Autodesk Fusion 360 part; units mm, degrees
(part 2 of 2)
  spline S168 degree 3 poles (-19.8203, 34.3524) (-19.856, 34.4918) (-19.8914, 34.6421) (-19.9257, 34.8034) knots 0 0 0 0 1 1 1 1
  spline S169 degree 3 poles (-19.9257, 34.8034) (-20.0542, 35.4074) (-20.1673, 36.1627) (-20.2205, 37.0718) knots 0 0 0 0 1 1 1 1
  arc A170 (-19.5901, 37.4087) -> (-20.2205, 37.0718) centre (0, 0) ccw
  spline S170 degree 3 poles (-19.5901, 37.4087) (-18.8638, 36.8595) (-18.2986, 36.3458) (-17.8679, 35.9033) knots 0 0 0 0 1 1 1 1
  spline S171 degree 3 poles (-17.8679, 35.9033) (-17.7528, 35.7852) (-17.6475, 35.6723) (-17.5514, 35.5652) knots 0 0 0 0 1 1 1 1
  arc A171 (-17.5514, 35.5652) -> (-17.0802, 35.472) centre (-17.2537, 35.8324) ccw
  arc A172 (-16.5847, 35.7064) -> (-17.0802, 35.472) centre (0, 0) ccw
  arc A173 (-16.5847, 35.7064) -> (-16.3578, 36.1297) centre (-16.7532, 36.0692) ccw
  spline S172 degree 3 poles (-16.3578, 36.1297) (-16.3796, 36.272) (-16.4, 36.425) (-16.4184, 36.5889) knots 0 0 0 0 1 1 1 1
  spline S173 degree 3 poles (-16.4184, 36.5889) (-16.4871, 37.2025) (-16.5257, 37.9653) (-16.4895, 38.8752) knots 0 0 0 0 1 1 1 1
  arc A174 (-15.8291, 39.1488) -> (-16.4895, 38.8752) centre (0, 0) ccw
  spline S174 degree 3 poles (-15.8291, 39.1488) (-15.1601, 38.531) (-14.648, 37.9643) (-14.2627, 37.4818) knots 0 0 0 0 1 1 1 1
  spline S175 degree 3 poles (-14.2627, 37.4818) (-14.1598, 37.353) (-14.0661, 37.2303) (-13.9809, 37.1143) knots 0 0 0 0 1 1 1 1
  arc A175 (-13.9809, 37.1143) -> (-13.5211, 36.9754) centre (-13.6585, 37.351) ccw
  arc A176 (-13.005, 37.16) -> (-13.5211, 36.9754) centre (0, 0) ccw
  arc A177 (-13.005, 37.16) -> (-12.7377, 37.5591) centre (-13.1371, 37.5376) ccw
  spline S176 degree 3 poles (-12.7377, 37.5591) (-12.7454, 37.7028) (-12.7508, 37.8571) (-12.753, 38.022) knots 0 0 0 0 1 1 1 1
  spline S177 degree 3 poles (-12.753, 38.022) (-12.7612, 38.6394) (-12.7248, 39.4023) (-12.5997, 40.3043) knots 0 0 0 0 1 1 1 1
  arc A178 (-11.9156, 40.5118) -> (-12.5997, 40.3043) centre (0, 0) ccw
  spline S178 degree 3 poles (-11.9156, 40.5118) (-11.3105, 39.8314) (-10.8563, 39.2173) (-10.5202, 38.6993) knots 0 0 0 0 1 1 1 1
  spline S179 degree 3 poles (-10.5202, 38.6993) (-10.4304, 38.561) (-10.3491, 38.4297) (-10.2757, 38.3059) knots 0 0 0 0 1 1 1 1
  arc A179 (-10.2757, 38.3059) -> (-9.8318, 38.1226) centre (-9.9317, 38.5099) ccw
  arc A180 (-9.3, 38.2558) -> (-9.8318, 38.1226) centre (0, 0) ccw
  arc A181 (-9.3, 38.2558) -> (-8.9949, 38.6267) centre (-9.3945, 38.6445) ccw
  spline S180 degree 3 poles (-8.9949, 38.6267) (-8.9885, 38.7705) (-8.9788, 38.9246) (-8.9648, 39.0889) knots 0 0 0 0 1 1 1 1
  spline S181 degree 3 poles (-8.9648, 39.0889) (-8.9125, 39.7042) (-8.8015, 40.4598) (-8.5885, 41.3452) knots 0 0 0 0 1 1 1 1
  arc A182 (-7.8874, 41.4846) -> (-8.5885, 41.3452) centre (0, 0) ccw
  spline S182 degree 3 poles (-7.8874, 41.4846) (-7.3518, 40.7482) (-6.9601, 40.0925) (-6.6763, 39.5441) knots 0 0 0 0 1 1 1 1
  spline S183 degree 3 poles (-6.6763, 39.5441) (-6.6005, 39.3977) (-6.5325, 39.259) (-6.4716, 39.1286) knots 0 0 0 0 1 1 1 1
  arc A183 (-6.4716, 39.1286) -> (-6.0478, 38.9027) centre (-6.1092, 39.298) ccw
  arc A184 (-5.5055, 38.9832) -> (-6.0478, 38.9027) centre (0, 0) ccw
  arc A185 (-5.5055, 38.9832) -> (-5.1655, 39.3224) centre (-5.5615, 39.3792) ccw
  spline S184 degree 3 poles (-5.1655, 39.3224) (-5.1451, 39.4649) (-5.1202, 39.6173) (-5.0902, 39.7794) knots 0 0 0 0 1 1 1 1
  spline S185 degree 3 poles (-5.0902, 39.7794) (-4.9779, 40.3866) (-4.7933, 41.1277) (-4.4946, 41.9879) knots 0 0 0 0 1 1 1 1
  arc A186 (-3.7832, 42.058) -> (-4.4946, 41.9879) centre (0, 0) ccw
  spline S186 degree 3 poles (-3.7832, 42.058) (-3.3224, 41.2726) (-2.9968, 40.5817) (-2.7682, 40.0081) knots 0 0 0 0 1 1 1 1
  spline S187 degree 3 poles (-2.7682, 40.0081) (-2.7071, 39.8549) (-2.653, 39.7103) (-2.6051, 39.5746) knots 0 0 0 0 1 1 1 1
  arc A187 (-2.6051, 39.5746) -> (-2.2055, 39.3082) centre (-2.2279, 39.7076) ccw
  arc A188 (-1.658, 39.3351) -> (-2.2055, 39.3082) centre (0, 0) ccw
  arc A189 (-1.658, 39.3351) -> (-1.2864, 39.6393) centre (-1.6748, 39.7347) ccw
  spline S188 degree 3 poles (-1.2864, 39.6393) (-1.2521, 39.7791) (-1.2124, 39.9284) (-1.1666, 40.0868) knots 0 0 0 0 1 1 1 1
  spline S189 degree 3 poles (-1.1666, 40.0868) (-0.9953, 40.68) (-0.739, 41.3995) (-0.3574, 42.2263) knots 0 0 0 0 1 1 1 1
  arc A190 (0.3574, 42.2263) -> (-0.3574, 42.2263) centre (0, 0) ccw
  spline S190 degree 3 poles (0.3574, 42.2263) (0.739, 41.3995) (0.9953, 40.68) (1.1666, 40.0868) knots 0 0 0 0 1 1 1 1
  spline S191 degree 3 poles (1.1666, 40.0868) (1.2124, 39.9284) (1.2521, 39.7791) (1.2864, 39.6393) knots 0 0 0 0 1 1 1 1
  arc A191 (1.2864, 39.6393) -> (1.658, 39.3351) centre (1.6748, 39.7347) ccw
  arc A192 (2.2055, 39.3082) -> (1.658, 39.3351) centre (0, 0) ccw
  arc A193 (2.2055, 39.3082) -> (2.6051, 39.5746) centre (2.2279, 39.7076) ccw
  spline S192 degree 3 poles (2.6051, 39.5746) (2.653, 39.7103) (2.7071, 39.8549) (2.7682, 40.0081) knots 0 0 0 0 1 1 1 1
  spline S193 degree 3 poles (2.7682, 40.0081) (2.9968, 40.5817) (3.3224, 41.2726) (3.7832, 42.058) knots 0 0 0 0 1 1 1 1
  arc A194 (4.4946, 41.9879) -> (3.7832, 42.058) centre (0, 0) ccw
  spline S194 degree 3 poles (4.4946, 41.9879) (4.7933, 41.1277) (4.9779, 40.3866) (5.0902, 39.7794) knots 0 0 0 0 1 1 1 1
  spline S195 degree 3 poles (5.0902, 39.7794) (5.1202, 39.6173) (5.1451, 39.4649) (5.1655, 39.3224) knots 0 0 0 0 1 1 1 1
  arc A195 (5.1655, 39.3224) -> (5.5055, 38.9832) centre (5.5615, 39.3792) ccw
  arc A196 (6.0478, 38.9027) -> (5.5055, 38.9832) centre (0, 0) ccw
  arc A197 (6.0478, 38.9027) -> (6.4716, 39.1286) centre (6.1092, 39.298) ccw
  spline S196 degree 3 poles (6.4716, 39.1286) (6.5325, 39.259) (6.6005, 39.3977) (6.6763, 39.5441) knots 0 0 0 0 1 1 1 1
  spline S197 degree 3 poles (6.6763, 39.5441) (6.9601, 40.0925) (7.3518, 40.7482) (7.8874, 41.4846) knots 0 0 0 0 1 1 1 1
  arc A198 (8.5885, 41.3452) -> (7.8874, 41.4846) centre (0, 0) ccw
  spline S198 degree 3 poles (8.5885, 41.3452) (8.8015, 40.4598) (8.9125, 39.7042) (8.9648, 39.0889) knots 0 0 0 0 1 1 1 1
  spline S199 degree 3 poles (8.9648, 39.0889) (8.9788, 38.9246) (8.9885, 38.7705) (8.9949, 38.6267) knots 0 0 0 0 1 1 1 1
  arc A199 (8.9949, 38.6267) -> (9.3, 38.2558) centre (9.3945, 38.6445) ccw
  arc A200 (9.8318, 38.1226) -> (9.3, 38.2558) centre (0, 0) ccw
  arc A201 (9.8318, 38.1226) -> (10.2757, 38.3059) centre (9.9317, 38.5099) ccw
  spline S200 degree 3 poles (10.2757, 38.3059) (10.3491, 38.4297) (10.4304, 38.561) (10.5202, 38.6993) knots 0 0 0 0 1 1 1 1
  spline S201 degree 3 poles (10.5202, 38.6993) (10.8563, 39.2173) (11.3105, 39.8314) (11.9156, 40.5118) knots 0 0 0 0 1 1 1 1
  arc A202 (12.5997, 40.3043) -> (11.9156, 40.5118) centre (0, 0) ccw
  spline S202 degree 3 poles (12.5997, 40.3043) (12.7248, 39.4023) (12.7612, 38.6394) (12.753, 38.022) knots 0 0 0 0 1 1 1 1
  spline S203 degree 3 poles (12.753, 38.022) (12.7508, 37.8571) (12.7454, 37.7028) (12.7377, 37.5591) knots 0 0 0 0 1 1 1 1
  arc A203 (12.7377, 37.5591) -> (13.005, 37.16) centre (13.1371, 37.5376) ccw
  arc A204 (13.5211, 36.9754) -> (13.005, 37.16) centre (0, 0) ccw
  arc A205 (13.5211, 36.9754) -> (13.9809, 37.1143) centre (13.6585, 37.351) ccw
  spline S204 degree 3 poles (13.9809, 37.1143) (14.0661, 37.2303) (14.1598, 37.353) (14.2627, 37.4818) knots 0 0 0 0 1 1 1 1
  spline S205 degree 3 poles (14.2627, 37.4818) (14.648, 37.9643) (15.1601, 38.531) (15.8291, 39.1488) knots 0 0 0 0 1 1 1 1
  arc A206 (16.4895, 38.8752) -> (15.8291, 39.1488) centre (0, 0) ccw
  spline S206 degree 3 poles (16.4895, 38.8752) (16.5257, 37.9653) (16.4871, 37.2025) (16.4184, 36.5889) knots 0 0 0 0 1 1 1 1
  spline S207 degree 3 poles (16.4184, 36.5889) (16.4, 36.425) (16.3796, 36.272) (16.3578, 36.1297) knots 0 0 0 0 1 1 1 1
  arc A207 (16.3578, 36.1297) -> (16.5847, 35.7064) centre (16.7532, 36.0692) ccw
  arc A208 (17.0802, 35.472) -> (16.5847, 35.7064) centre (0, 0) ccw
  arc A209 (17.0802, 35.472) -> (17.5514, 35.5652) centre (17.2537, 35.8324) ccw
  spline S208 degree 3 poles (17.5514, 35.5652) (17.6475, 35.6723) (17.7528, 35.7852) (17.8679, 35.9033) knots 0 0 0 0 1 1 1 1
  spline S209 degree 3 poles (17.8679, 35.9033) (18.2986, 36.3458) (18.8638, 36.8595) (19.5901, 37.4087) knots 0 0 0 0 1 1 1 1
  arc A210 (20.2205, 37.0718) -> (19.5901, 37.4087) centre (0, 0) ccw
  spline S210 degree 3 poles (20.2205, 37.0718) (20.1673, 36.1627) (20.0542, 35.4074) (19.9257, 34.8034) knots 0 0 0 0 1 1 1 1
  spline S211 degree 3 poles (19.9257, 34.8034) (19.8914, 34.6421) (19.856, 34.4918) (19.8203, 34.3524) knots 0 0 0 0 1 1 1 1
  arc A211 (19.8203, 34.3524) -> (20.0046, 33.9089) centre (20.2079, 34.2534) ccw
  arc A212 (20.4748, 33.6271) -> (20.0046, 33.9089) centre (0, 0) ccw
  arc A213 (20.4748, 33.6271) -> (20.9528, 33.6736) centre (20.6829, 33.9687) ccw
  spline S212 degree 3 poles (20.9528, 33.6736) (21.0591, 33.7707) (21.1749, 33.8728) (21.301, 33.9791) knots 0 0 0 0 1 1 1 1
  spline S213 degree 3 poles (21.301, 33.9791) (21.773, 34.3772) (22.3859, 34.833) (23.1625, 35.3084) knots 0 0 0 0 1 1 1 1
  arc A214 (23.7568, 34.9113) -> (23.1625, 35.3084) centre (0, 0) ccw
  spline S214 degree 3 poles (23.7568, 34.9113) (23.6148, 34.0119) (23.4282, 33.2712) (23.2411, 32.6828) knots 0 0 0 0 1 1 1 1
  spline S215 degree 3 poles (23.2411, 32.6828) (23.1911, 32.5256) (23.1411, 32.3795) (23.092, 32.2442) knots 0 0 0 0 1 1 1 1
  arc A215 (23.092, 32.2442) -> (23.232, 31.7848) centre (23.468, 32.1077) ccw
  arc A216 (23.6723, 31.4583) -> (23.232, 31.7848) centre (0, 0) ccw
  arc A217 (23.6723, 31.4583) -> (24.1525, 31.4577) centre (23.9128, 31.7779) ccw
  spline S216 degree 3 poles (24.1525, 31.4577) (24.2678, 31.544) (24.3931, 31.6342) (24.529, 31.7276) knots 0 0 0 0 1 1 1 1
  spline S217 degree 3 poles (24.529, 31.7276) (25.0377, 32.0775) (25.6923, 32.4711) (26.5118, 32.8681) knots 0 0 0 0 1 1 1 1
  arc A218 (27.0644, 32.4146) -> (26.5118, 32.8681) centre (0, 0) ccw
  spline S218 degree 3 poles (27.0644, 32.4146) (26.8348, 31.5334) (26.5765, 30.8146) (26.3326, 30.2474) knots 0 0 0 0 1 1 1 1
  spline S219 degree 3 poles (26.3326, 30.2474) (26.2675, 30.0959) (26.2035, 29.9554) (26.1413, 29.8255) knots 0 0 0 0 1 1 1 1
  arc A219 (26.1413, 29.8255) -> (26.2356, 29.3546) centre (26.5021, 29.6529) ccw
  arc A220 (26.6417, 28.9865) -> (26.2356, 29.3546) centre (0, 0) ccw
  arc A221 (26.6417, 28.9865) -> (27.1196, 28.9389) centre (26.9124, 29.281) ccw
  spline S220 degree 3 poles (27.1196, 28.9389) (27.2428, 29.0134) (27.3763, 29.0909) (27.5207, 29.1706) knots 0 0 0 0 1 1 1 1
  spline S221 degree 3 poles (27.5207, 29.1706) (28.0613, 29.4689) (28.7513, 29.7964) (29.6058, 30.1112) knots 0 0 0 0 1 1 1 1
  arc A222 (30.1112, 29.6058) -> (29.6058, 30.1112) centre (0, 0) ccw
  spline S222 degree 3 poles (30.1112, 29.6058) (29.7964, 28.7513) (29.4689, 28.0613) (29.1706, 27.5207) knots 0 0 0 0 1 1 1 1
  spline S223 degree 3 poles (29.1706, 27.5207) (29.0909, 27.3763) (29.0134, 27.2428) (28.9389, 27.1196) knots 0 0 0 0 1 1 1 1
  arc A223 (28.9389, 27.1196) -> (28.9865, 26.6417) centre (29.281, 26.9124) ccw
  arc A224 (29.3546, 26.2356) -> (28.9865, 26.6417) centre (0, 0) ccw
  arc A225 (29.3546, 26.2356) -> (29.8255, 26.1413) centre (29.6529, 26.5021) ccw
  spline S224 degree 3 poles (29.8255, 26.1413) (29.9554, 26.2035) (30.0959, 26.2675) (30.2474, 26.3326) knots 0 0 0 0 1 1 1 1
  spline S225 degree 3 poles (30.2474, 26.3326) (30.8146, 26.5765) (31.5334, 26.8348) (32.4146, 27.0644) knots 0 0 0 0 1 1 1 1
  arc A226 (32.8681, 26.5118) -> (32.4146, 27.0644) centre (0, 0) ccw
  spline S226 degree 3 poles (32.8681, 26.5118) (32.4711, 25.6923) (32.0775, 25.0377) (31.7276, 24.529) knots 0 0 0 0 1 1 1 1
  spline S227 degree 3 poles (31.7276, 24.529) (31.6342, 24.3931) (31.544, 24.2678) (31.4577, 24.1525) knots 0 0 0 0 1 1 1 1
  arc A227 (31.4577, 24.1525) -> (31.4583, 23.6723) centre (31.7779, 23.9128) ccw
  arc A228 (31.7848, 23.232) -> (31.4583, 23.6723) centre (0, 0) ccw
  arc A229 (31.7848, 23.232) -> (32.2442, 23.092) centre (32.1077, 23.468) ccw
  spline S228 degree 3 poles (32.2442, 23.092) (32.3795, 23.1411) (32.5256, 23.1911) (32.6828, 23.2411) knots 0 0 0 0 1 1 1 1
  spline S229 degree 3 poles (32.6828, 23.2411) (33.2712, 23.4282) (34.0119, 23.6148) (34.9113, 23.7568) knots 0 0 0 0 1 1 1 1
  arc A230 (35.3084, 23.1625) -> (34.9113, 23.7568) centre (0, 0) ccw
  spline S230 degree 3 poles (35.3084, 23.1625) (34.833, 22.3859) (34.3772, 21.773) (33.9791, 21.301) knots 0 0 0 0 1 1 1 1
  spline S231 degree 3 poles (33.9791, 21.301) (33.8728, 21.1749) (33.7707, 21.0591) (33.6736, 20.9528) knots 0 0 0 0 1 1 1 1
  arc A231 (33.6736, 20.9528) -> (33.6271, 20.4748) centre (33.9687, 20.6829) ccw
  arc A232 (33.9089, 20.0046) -> (33.6271, 20.4748) centre (0, 0) ccw
  arc A233 (33.9089, 20.0046) -> (34.3524, 19.8203) centre (34.2534, 20.2079) ccw
  spline S232 degree 3 poles (34.3524, 19.8203) (34.4918, 19.856) (34.6421, 19.8914) (34.8034, 19.9257) knots 0 0 0 0 1 1 1 1
  spline S233 degree 3 poles (34.8034, 19.9257) (35.4074, 20.0542) (36.1627, 20.1673) (37.0718, 20.2205) knots 0 0 0 0 1 1 1 1
  arc A234 (37.4087, 19.5901) -> (37.0718, 20.2205) centre (0, 0) ccw
  spline S234 degree 3 poles (37.4087, 19.5901) (36.8595, 18.8638) (36.3458, 18.2986) (35.9033, 17.8679) knots 0 0 0 0 1 1 1 1
  spline S235 degree 3 poles (35.9033, 17.8679) (35.7852, 17.7528) (35.6723, 17.6475) (35.5652, 17.5514) knots 0 0 0 0 1 1 1 1
  arc A235 (35.5652, 17.5514) -> (35.472, 17.0802) centre (35.8324, 17.2537) ccw
  arc A236 (35.7064, 16.5847) -> (35.472, 17.0802) centre (0, 0) ccw
  arc A237 (35.7064, 16.5847) -> (36.1297, 16.3578) centre (36.0692, 16.7532) ccw
  spline S236 degree 3 poles (36.1297, 16.3578) (36.272, 16.3796) (36.425, 16.4) (36.5889, 16.4184) knots 0 0 0 0 1 1 1 1
  spline S237 degree 3 poles (36.5889, 16.4184) (37.2025, 16.4871) (37.9653, 16.5257) (38.8752, 16.4895) knots 0 0 0 0 1 1 1 1
  arc A238 (39.1488, 15.8291) -> (38.8752, 16.4895) centre (0, 0) ccw
  spline S238 degree 3 poles (39.1488, 15.8291) (38.531, 15.1601) (37.9643, 14.648) (37.4818, 14.2627) knots 0 0 0 0 1 1 1 1
  spline S239 degree 3 poles (37.4818, 14.2627) (37.353, 14.1598) (37.2303, 14.0661) (37.1143, 13.9809) knots 0 0 0 0 1 1 1 1
  arc A239 (37.1143, 13.9809) -> (36.9754, 13.5211) centre (37.351, 13.6585) ccw
  arc A240 (37.16, 13.005) -> (36.9754, 13.5211) centre (0, 0) ccw
  arc A241 (37.16, 13.005) -> (37.5591, 12.7377) centre (37.5376, 13.1371) ccw
  spline S240 degree 3 poles (37.5591, 12.7377) (37.7028, 12.7454) (37.8571, 12.7508) (38.022, 12.753) knots 0 0 0 0 1 1 1 1
  spline S241 degree 3 poles (38.022, 12.753) (38.6394, 12.7612) (39.4023, 12.7248) (40.3043, 12.5997) knots 0 0 0 0 1 1 1 1
  arc A242 (40.5118, 11.9156) -> (40.3043, 12.5997) centre (0, 0) ccw
  spline S242 degree 3 poles (40.5118, 11.9156) (39.8314, 11.3105) (39.2173, 10.8563) (38.6993, 10.5202) knots 0 0 0 0 1 1 1 1
  spline S243 degree 3 poles (38.6993, 10.5202) (38.561, 10.4304) (38.4297, 10.3491) (38.3059, 10.2757) knots 0 0 0 0 1 1 1 1
  arc A243 (38.3059, 10.2757) -> (38.1226, 9.8318) centre (38.5099, 9.9317) ccw
  arc A244 (38.2558, 9.3) -> (38.1226, 9.8318) centre (0, 0) ccw
  arc A245 (38.2558, 9.3) -> (38.6267, 8.9949) centre (38.6445, 9.3945) ccw
  spline S244 degree 3 poles (38.6267, 8.9949) (38.7705, 8.9885) (38.9246, 8.9788) (39.0889, 8.9648) knots 0 0 0 0 1 1 1 1
  spline S245 degree 3 poles (39.0889, 8.9648) (39.7042, 8.9125) (40.4598, 8.8015) (41.3452, 8.5885) knots 0 0 0 0 1 1 1 1
  arc A246 (41.4846, 7.8874) -> (41.3452, 8.5885) centre (0, 0) ccw
  spline S246 degree 3 poles (41.4846, 7.8874) (40.7482, 7.3518) (40.0925, 6.9601) (39.5441, 6.6763) knots 0 0 0 0 1 1 1 1
  spline S247 degree 3 poles (39.5441, 6.6763) (39.3977, 6.6005) (39.259, 6.5325) (39.1286, 6.4716) knots 0 0 0 0 1 1 1 1
  arc A247 (39.1286, 6.4716) -> (38.9027, 6.0478) centre (39.298, 6.1092) ccw
  arc A248 (38.9832, 5.5055) -> (38.9027, 6.0478) centre (0, 0) ccw
  arc A249 (38.9832, 5.5055) -> (39.3224, 5.1655) centre (39.3792, 5.5615) ccw
  spline S248 degree 3 poles (39.3224, 5.1655) (39.4649, 5.1451) (39.6173, 5.1202) (39.7794, 5.0902) knots 0 0 0 0 1 1 1 1
  spline S249 degree 3 poles (39.7794, 5.0902) (40.3866, 4.9779) (41.1277, 4.7933) (41.9879, 4.4946) knots 0 0 0 0 1 1 1 1
  arc A250 (42.058, 3.7832) -> (41.9879, 4.4946) centre (0, 0) ccw
  spline S250 degree 3 poles (42.058, 3.7832) (41.2726, 3.3224) (40.5817, 2.9968) (40.0081, 2.7682) knots 0 0 0 0 1 1 1 1
  spline S251 degree 3 poles (40.0081, 2.7682) (39.8549, 2.7071) (39.7103, 2.653) (39.5746, 2.6051) knots 0 0 0 0 1 1 1 1
  arc A251 (39.5746, 2.6051) -> (39.3082, 2.2055) centre (39.7076, 2.2279) ccw
  arc A252 (39.3351, 1.658) -> (39.3082, 2.2055) centre (0, 0) ccw
  arc A253 (39.3351, 1.658) -> (39.6393, 1.2864) centre (39.7347, 1.6748) ccw
  spline S252 degree 3 poles (39.6393, 1.2864) (39.7791, 1.2521) (39.9284, 1.2124) (40.0868, 1.1666) knots 0 0 0 0 1 1 1 1
  spline S253 degree 3 poles (40.0868, 1.1666) (40.68, 0.9953) (41.3995, 0.739) (42.2263, 0.3574) knots 0 0 0 0 1 1 1 1
  arc A254 (42.2263, -0.3574) -> (42.2263, 0.3574) centre (0, 0) ccw
  spline S254 degree 3 poles (42.2263, -0.3574) (41.3995, -0.739) (40.68, -0.9953) (40.0868, -1.1666) knots 0 0 0 0 1 1 1 1
  spline S255 degree 3 poles (40.0868, -1.1666) (39.9284, -1.2124) (39.7791, -1.2521) (39.6393, -1.2864) knots 0 0 0 0 1 1 1 1
  arc A255 (39.6393, -1.2864) -> (39.3351, -1.658) centre (39.7347, -1.6748) ccw
  arc A256 (39.3082, -2.2055) -> (39.3351, -1.658) centre (0, 0) ccw
extrude "Extrude1'" add sketch "Sketch1 (2)" along normal blind 20 separate body makes body 2 in component "Internal Gear (64 teeth)"
sketch "Sketch2 (2)" plane through (0, 0, 0) normal (0, 1, 0) x (1, 0, 0) in component "Internal Gear (64 teeth)"
  circle A0 centre (0, 0) radius 40.64 construction
sketch "Sketch7" plane through (0, 0, 10) normal (0, 0, 1) x (-1, 0, 0)
sketch "Sketch5" plane through (0, 0, 10) normal (0, 0, 1) x (-1, 0, 0)
combine "Combine1" operation add target body 1 tool bodies 2 body 2 seen with x (0, 1, 0) y (0, 0, 1) z (1, 0, 0) at (0.1776, -0.0314, 9.9576)
sketch "Sketch10" plane through (0, 0, 30) normal (0, 0, 1) x (-1, 0, 0)
  circle A0 centre (0, 0) radius 25
  circle A1 centre (0, 0) radius 11.5
  dimension "d39" = 23
  constraint concentric A0 A1
  measures "d39" diameter of A1
extrude "Extrude4" cut sketch "Sketch10" against normal blind 8 contours A1 bodies 1
sketch "Sketch11" plane through (0, 0, 0) normal (0, 0, -1) x (1, 0, 0)
  line L0 (-11.2871, -94.6657) -> (-26.9596, -91.445)
  line L1 (-26.9596, -91.445) -> (-19.995, -72.4583)
  line L2 (-19.995, -72.4583) -> (-10.1997, -74.4712)
  line L3 (-10.1997, -74.4712) -> (-11.2871, -94.6657)
  line L4 (-76.3895, -57.0407) -> (-84.8529, -43.4624)
  line L5 (-84.8529, -43.4624) -> (-66.2931, -35.4291)
  line L6 (-66.2931, -35.4291) -> (-61.0035, -43.9155)
  line L7 (-61.0035, -43.9155) -> (-76.3895, -57.0407)
  line L8 (-93.9725, 16.0674) -> (-89.9621, 31.5566)
  line L9 (-89.9621, 31.5566) -> (-71.3525, 23.6393)
  line L10 (-71.3525, 23.6393) -> (-73.859, 13.9586)
  line L11 (-73.859, 13.9586) -> (-93.9725, 16.0674)
  line L12 (-53.0985, 79.1805) -> (-39.1089, 86.9453)
  line L13 (-39.1089, 86.9453) -> (-32.0259, 68.0025)
  line L14 (-32.0259, 68.0025) -> (-40.7694, 63.1495)
  line L15 (-40.7694, 63.1495) -> (-53.0985, 79.1805)
  line L16 (20.8064, 93.0381) -> (36.0726, 88.2483)
  line L17 (36.0726, 88.2483) -> (27.2229, 70.0636)
  line L18 (27.2229, 70.0636) -> (17.6815, 73.0573)
  line L19 (17.6815, 73.0573) -> (20.8064, 93.0381)
  line L20 (81.7683, 49.0199) -> (88.8146, 34.655)
  line L21 (88.8146, 34.655) -> (69.5373, 28.5405)
  line L22 (69.5373, 28.5405) -> (65.1334, 37.5186)
  line L23 (65.1334, 37.5186) -> (81.7683, 49.0199)
  line L24 (91.8649, -25.492) -> (86.308, -40.496)
  line L25 (86.308, -40.496) -> (68.5949, -30.7367)
  line L26 (68.5949, -30.7367) -> (72.0679, -21.3591)
  line L27 (72.0679, -21.3591) -> (91.8649, -25.492)
  line L28 (60.8366, -73.4024) -> (47.7044, -82.5427)
  line L29 (47.7044, -82.5427) -> (38.7413, -64.4136)
  line L30 (38.7413, -64.4136) -> (46.9489, -58.7009)
  line L31 (46.9489, -58.7009) -> (60.8366, -73.4024)
  line L32 (95.1159, -6.4779) -> (92.6931, -22.2934)
  line L33 (92.6931, -22.2934) -> (73.378, -16.2994)
  line L34 (73.378, -16.2994) -> (74.8923, -6.4147)
  line L35 (74.8923, -6.4147) -> (95.1159, -6.4779)
  line L36 (70.2268, 64.4763) -> (80.0205, 51.8239)
  line L37 (80.0205, 51.8239) -> (62.3687, 41.9541)
  line L38 (62.3687, 41.9541) -> (56.2477, 49.8618)
  line L39 (56.2477, 49.8618) -> (70.2268, 64.4763)
  line L40 (1.652, 95.3219) -> (17.5699, 93.7032)
  line L41 (17.5699, 93.7032) -> (12.562, 74.1094)
  line L42 (12.562, 74.1094) -> (2.6133, 75.121)
  line L43 (2.6133, 75.121) -> (1.652, 95.3219)
  line L44 (-67.9505, 66.871) -> (-55.8103, 77.293)
  line L45 (-55.8103, 77.293) -> (-45.0591, 60.1637)
  line L46 (-45.0591, 60.1637) -> (-52.6467, 53.65)
  line L47 (-52.6467, 53.65) -> (-67.9505, 66.871)
  line L48 (-95.2833, -3.1781) -> (-94.4729, 12.8014)
  line L49 (-94.4729, 12.8014) -> (-74.6505, 8.7923)
  line L50 (-74.6505, 8.7923) -> (-75.157, -1.1949)
  line L51 (-75.157, -1.1949) -> (-95.2833, -3.1781)
  line L52 (-63.3436, -71.2502) -> (-74.3671, -59.6535)
  line L53 (-74.3671, -59.6535) -> (-57.8043, -48.0486)
  line L54 (-57.8043, -48.0486) -> (-50.9146, -55.2965)
  line L55 (-50.9146, -55.2965) -> (-63.3436, -71.2502)
  line L56 (5, -75) -> (8, -95)
  line L57 (8, -95) -> (-8, -95)
  line L58 (-8, -95) -> (-5, -75)
  line L59 (-5, -75) -> (5, -75)
  line L60 (-30.1121, -90.4558) -> (-44.8155, -84.1461)
  line L61 (-44.8155, -84.1461) -> (-34.1715, -66.9501)
  line L62 (-34.1715, -66.9501) -> (-24.9819, -70.8936)
  line L63 (-24.9819, -70.8936) -> (-30.1121, -90.4558)
  line L64 (-86.308, -40.496) -> (-91.8649, -25.492)
  line L65 (-91.8649, -25.492) -> (-72.0679, -21.3591)
  line L66 (-72.0679, -21.3591) -> (-68.5949, -30.7367)
  line L67 (-68.5949, -30.7367) -> (-86.308, -40.496)
  line L68 (-88.8146, 34.655) -> (-81.7683, 49.0199)
  line L69 (-81.7683, 49.0199) -> (-65.1334, 37.5186)
  line L70 (-65.1334, 37.5186) -> (-69.5373, 28.5405)
  line L71 (-69.5373, 28.5405) -> (-88.8146, 34.655)
  line L72 (-36.0726, 88.2483) -> (-20.8064, 93.0381)
  line L73 (-20.8064, 93.0381) -> (-17.6815, 73.0573)
  line L74 (-17.6815, 73.0573) -> (-27.2229, 70.0636)
  line L75 (-27.2229, 70.0636) -> (-36.0726, 88.2483)
  line L76 (39.1089, 86.9453) -> (53.0985, 79.1805)
  line L77 (53.0985, 79.1805) -> (40.7694, 63.1495)
  line L78 (40.7694, 63.1495) -> (32.0259, 68.0025)
  line L79 (32.0259, 68.0025) -> (39.1089, 86.9453)
  line L80 (89.9621, 31.5566) -> (93.9725, 16.0674)
  line L81 (93.9725, 16.0674) -> (73.859, 13.9586)
  line L82 (73.859, 13.9586) -> (71.3525, 23.6393)
  line L83 (71.3525, 23.6393) -> (89.9621, 31.5566)
  line L84 (84.8529, -43.4624) -> (76.3895, -57.0407)
  line L85 (76.3895, -57.0407) -> (61.0035, -43.9155)
  line L86 (61.0035, -43.9155) -> (66.2931, -35.4291)
  line L87 (66.2931, -35.4291) -> (84.8529, -43.4624)
  line L88 (74.3671, -59.6535) -> (63.3436, -71.2502)
  line L89 (63.3436, -71.2502) -> (50.9146, -55.2965)
  line L90 (50.9146, -55.2965) -> (57.8043, -48.0486)
  line L91 (57.8043, -48.0486) -> (74.3671, -59.6535)
  line L92 (94.4729, 12.8014) -> (95.2833, -3.1781)
  line L93 (95.2833, -3.1781) -> (75.157, -1.1949)
  line L94 (75.157, -1.1949) -> (74.6505, 8.7923)
  line L95 (74.6505, 8.7923) -> (94.4729, 12.8014)
  line L96 (55.8103, 77.293) -> (67.9505, 66.871)
  line L97 (67.9505, 66.871) -> (52.6467, 53.65)
  line L98 (52.6467, 53.65) -> (45.0591, 60.1637)
  line L99 (45.0591, 60.1637) -> (55.8103, 77.293)
  line L100 (-17.5699, 93.7032) -> (-1.652, 95.3219)
  line L101 (-1.652, 95.3219) -> (-2.6133, 75.121)
  line L102 (-2.6133, 75.121) -> (-12.562, 74.1094)
  line L103 (-12.562, 74.1094) -> (-17.5699, 93.7032)
  line L104 (-80.0205, 51.8239) -> (-70.2268, 64.4763)
  line L105 (-70.2268, 64.4763) -> (-56.2477, 49.8618)
  line L106 (-56.2477, 49.8618) -> (-62.3687, 41.9541)
  line L107 (-62.3687, 41.9541) -> (-80.0205, 51.8239)
  line L108 (-92.6931, -22.2934) -> (-95.1159, -6.4779)
  line L109 (-95.1159, -6.4779) -> (-74.8923, -6.4147)
  line L110 (-74.8923, -6.4147) -> (-73.378, -16.2994)
  line L111 (-73.378, -16.2994) -> (-92.6931, -22.2934)
  line L112 (-47.7044, -82.5427) -> (-60.8366, -73.4024)
  line L113 (-60.8366, -73.4024) -> (-46.9489, -58.7009)
  line L114 (-46.9489, -58.7009) -> (-38.7413, -64.4136)
  line L115 (-38.7413, -64.4136) -> (-47.7044, -82.5427)
  line L116 (26.9596, -91.445) -> (11.2871, -94.6657)
  line L117 (11.2871, -94.6657) -> (10.1997, -74.4712)
  line L118 (10.1997, -74.4712) -> (19.995, -72.4583)
  line L119 (19.995, -72.4583) -> (26.9596, -91.445)
  circle A0 centre (0, 0) radius 100
  circle A1 centre (0, 0) radius 11.5
  dimension "d42" = 23
  constraint coincident A0.centre A1.centre
  measures "d42" diameter of A1
extrude "Extrude5" cut sketch "Sketch11" against normal blind 8 contours A1 bodies 1
sketch "Sketch12" plane through (0, 0, 22) normal (0, 0, 1) x (-1, 0, 0)
  circle A0 centre (0, 0) radius 11.5
  circle A1 centre (0, 0) radius 5
  dimension "d45" = 10
  constraint coincident A0.centre A1.centre
  measures "d45" diameter of A1
extrude "Extrude6" cut sketch "Sketch12" against normal blind 20 contours A1 bodies 1
component "Internal Gear (64 teeth)" placed x (0, 1, 0) y (0, 0, 1) z (1, 0, 0) at (0.1776, -0.0314, 9.9576)
equation "disc_diameter = 200 mm"
equation "disc_height = 30 mm"
equation "d3 = disc_diameter"
equation "d4 = disc_height"
equation "hole_depth = -30 mm"
equation "d9 = hole_depth"
equation "tooth_ring = 90 mm"
equation "d12 = tooth_ring"
equation "tooth_ring_inner = 50 mm"
equation "d14 = tooth_ring_inner"
equation "tooth_ring_depth = -20 mm"
equation "d16 = tooth_ring_depth"
equation "center_hole = 10 mm"
equation "bearing_dia = 23 mm"
equation "bearing_height = -8 mm"
equation "shaft_hole = 10 mm"
equation "shaft_hole_lenth = -20 mm"
equation "d39 = bearing_dia"
equation "d40 = bearing_height"
equation "d42 = bearing_dia"
equation "d43 = bearing_height"
equation "d45 = shaft_hole"
equation "d46 = shaft_hole_lenth"
